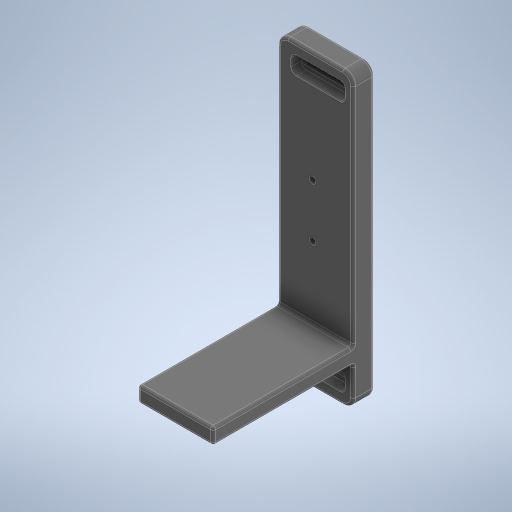
# Autodesk Inventor part: defmormable mirror mount
Saved by Autodesk Inventor 2023 (Build 270158030, 158C)
## iProperties
Created: 2025-06-09
Part Number: defmormable mirror mount
Material: Generisch
Document SubType Name: Modeling
Designer: Julian
Density: 1 g/cm^3
Appearance: Vorgabe
Author: Julian
Autodesk Inventor part; units mm, degrees
ref_plane "YZ Plane" through (0, 0, 0) normal (1, 0, 0) x (0, 1, 0)
ref_plane "XZ Plane" through (0, 0, 0) normal (0, 1, 0) x (-1, 0, 0)
ref_plane "XY Plane" through (0, 0, 0) normal (0, 0, 1) x (1, 0, 0)
sketch "Skizze1" plane through (0, 0, 0) normal (0, 0, 1) x (1, 0, 0)
  circle A0 centre (-10.43, 42) radius 1.25
  circle A1 centre (-10.43, 22) radius 1.25
  line L0 (-18.6, 59) -> (0, 59)
  line L1 (0, 59) -> (0, 0)
  line L2 (-18.6, 0) -> (0, 0)
  line L3 (-18.6, 0) -> (-18.6, 59)
  line L4 (-18.6, 0) -> (-18.6, -5)
  line L5 (0, -5) -> (-18.6, -5)
  line L6 (0, -5) -> (0, 0)
  line L7 (0, 59) -> (0, 69)
  line L8 (-18.6, 69) -> (0, 69)
  line L9 (-18.6, 69) -> (-18.6, 59)
  line L10 (-18.6, 69) -> (-23.6, 69)
  line L11 (-23.6, 69) -> (-23.6, 84)
  line L12 (-23.6, 84) -> (-18.6, 84)
  line L13 (-18.6, 84) -> (-18.6, 69)
  line L14 (-23.6, 84) -> (5, 84)
  line L15 (5, 84) -> (5, -26)
  line L16 (5, -26) -> (-23.6, -26)
  line L17 (-23.6, -26) -> (-23.6, 84)
  line L18 (5, -5) -> (-23.6, -5)
  line L19 (-23.6, -5) -> (-23.6, -11)
  line L20 (-23.6, -11) -> (5, -11)
  line L21 (5, -11) -> (5, -5)
  line L22 (5, 84) -> (2, 84)
  line L23 (2, 84) -> (2, 80)
  line L24 (2, 80) -> (5, 80)
  line L25 (5, 80) -> (5, 84)
  line L26 (2, 80) -> (-20.6, 80)
  line L27 (-20.6, 80) -> (-20.6, 73)
  line L28 (-20.6, 73) -> (2, 73)
  line L29 (2, 73) -> (2, 80)
  line L30 (5, -11) -> (2, -11)
  line L31 (2, -11) -> (2, -15)
  line L32 (2, -15) -> (5, -15)
  line L33 (5, -15) -> (5, -11)
  line L34 (2, -15) -> (-20.6, -15)
  line L35 (-20.6, -15) -> (-20.6, -22)
  line L36 (-20.6, -22) -> (2, -22)
  line L37 (2, -22) -> (2, -15)
  line L38 (-20.6, 80) -> (-19.1, 80)
  line L39 (-19.1, 80) -> (-19.1, 78.5)
  line L40 (-19.1, 78.5) -> (-20.6, 78.5)
  line L41 (-20.6, 78.5) -> (-20.6, 80)
  line L42 (-19.1, 78.311) -> (0.5, 78.311)
  line L43 (0.5, 78.311) -> (0.5, 74.311)
  line L44 (0.5, 74.311) -> (-19.1, 74.311)
  line L45 (-19.1, 74.311) -> (-19.1, 78.311)
  line L46 (-20.6, -15) -> (-19.1, -15)
  line L47 (-19.1, -15) -> (-19.1, -16.5)
  line L48 (-19.1, -16.5) -> (-20.6, -16.5)
  line L49 (-20.6, -16.5) -> (-20.6, -15)
  line L50 (-19.1, -16.5) -> (0.5, -16.5)
  line L51 (0.5, -16.5) -> (0.5, -20.5)
  line L52 (0.5, -20.5) -> (-19.1, -20.5)
  line L53 (-19.1, -20.5) -> (-19.1, -16.5)
  point P0 (0, 32)
  point P1 (-18.6, 80)
  point P2 (-18.6, 73)
  point P3 (-18.6, 78.311)
  point P4 (-18.6, 74.311)
  dimension "d0" = 5
  dimension "d1" = 15
  dimension "d2" = 28.6
  dimension "d3" = 110
  dimension "d4" = 6
  dimension "d5" = 3
  dimension "d6" = 4
  dimension "d7" = 22.6
  dimension "d8" = 7
  dimension "d9" = 3
  dimension "d10" = 4
  dimension "d11" = 22.6
  dimension "d12" = 7
  dimension "d22" = 1.5
  dimension "d23" = 1.5
  dimension "d24" = 19.6
  dimension "d25" = 4
  dimension "d26" = 1.5
  dimension "d27" = 1.5
  dimension "d28" = 4
  constraints: 108 end point, 22 parallel, 11 horizontal, 11 perpendicular, 4 point on line, 2 centre point
  measures "d0" distance of L11.end L12.end
  measures "d1" distance of L10.end L11.end
  measures "d2" distance of L15.end L16.end
  measures "d3" distance of L14.end L15.end
  measures "d4" distance of L19.end L18.end
  measures "d5" distance of L24.end L23.end
  measures "d6" distance of L23.end L22.end
  measures "d7" distance of L28.end L27.end
  measures "d8" distance of L27.end L26.end
  measures "d9" distance of L32.end L31.end
  measures "d10" distance of L31.end L30.end
  measures "d11" distance of L36.end L35.end
  measures "d12" distance of L35.end L34.end
  measures "d22" distance of L39.end L40.end
  measures "d23" distance of L38.end L39.end
  measures "d24" distance of L43.end L44.end
  measures "d25" distance of L42.end L43.end
  measures "d26" distance of L47.end L48.end
  measures "d27" distance of L46.end L47.end
  measures "d28" distance of L50.end L51.end
extrude "Extrusion1" add sketch "Skizze1" along normal blind 4 contours L13 L44 L43 L42 L26 L29 L28 | L37 L36 L35 L48 L47 L34 | L47 L48 L35 L34
extrude "Extrusion2" add sketch "Skizze1" along normal blind 8 contours L9 L8 L7 L0 | L0 L1 L2 L3 | L3 L4 L18 L17 L10 L9 | L7 L8 L13 L28 L29 L24 L15 L18 L6 L1 | L2 L6 L5 L4 | L10 L11 L12 L13 L26 L27 L28 | L5 L18 L15 L20 L17 | L28 L27 L40 L39 L26 L13 L42 L45 L44 | L44 L45 L42 L13 | L20 L31 L32 L15 L16 L17 | L14 L23 L26 L13 | L27 L26 L39 L40 | L23 L14 L15 L24 | L15 L32 L31 L20
extrude "Extrusion3" add sketch "Skizze1" along normal blind 61 contours L5 L18 L15 L20 L17
fillet "Rundung1" radius 4 4 edges at (5, -26, 4) (-23.6, -26, 4) (5, 84, 4) (-23.6, 84, 4)
fillet "Rundung2" radius 1 27 edges at (-22.4284, 82.8284, 0) (-23.6, 29, 0) (-22.4284, -24.8284, 0) (-9.3, -26, 0) (3.8284, -24.8284, 0) (5, 29, 0) (3.8284, 82.8284, 0) (-9.3, 84, 0) (-22.4284, 82.8284, 8) (-23.6, 37.5, 8) (3.8284, 82.8284, 8) (5, 37.5, 8) (-9.3, 84, 8) (3.8284, -24.8284, 8) (5, -16.5, 8) (-22.4284, -24.8284, 8) (-9.3, -26, 8) (5, -8, 61) (-9.3, -5, 8) (-9.3, -11, 8) (5, -11, 34.5) (5, -5, 34.5) (-23.6, -8, 61) (-9.3, -5, 61) (-9.3, -11, 61) (-23.6, -5, 34.5) (-23.6, -11, 34.5)
fillet "Rundung3" radius 2 8 edges at (-20.6, -22, 6) (-20.6, -15, 6) (2, -15, 6) (2, -22, 6) (-18.6, 73, 6) (-18.6, 80, 6) (2, 80, 6) (2, 73, 6)
fillet "Rundung4" radius 1 8 edges at (-18.5757, 78.311, 2) (-18.4776, 74.311, 2) (0.5, 74.311, 2) (0.5, 78.311, 2) (-19.1, -20.5, 2) (-19.1, -16.5, 2) (0.5, -20.5, 2) (0.5, -16.5, 2)
